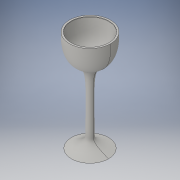
# Autodesk Inventor part: Wine Glass Placeholder
Saved by Autodesk Inventor 2016 (Build 200138000, 138)
## iProperties
Created: 2017-10-31
Part Number: Wine Glass Placeholder
Material: Generic
Document SubType Name: Modeling
Designer: mathaetaes
Density: 1 g/cm^3
Appearance: Default
Author: mathaetaes
Autodesk Inventor part; units mm, degrees
ref_plane "YZ Plane" through (0, 0, 0) normal (1, 0, 0) x (0, 1, 0)
ref_plane "XZ Plane" through (0, 0, 0) normal (0, 1, 0) x (-1, 0, 0)
ref_plane "XY Plane" through (0, 0, 0) normal (0, 0, 1) x (1, 0, 0)
sketch "Sketch2" plane through (0, 0, 0) normal (0, 0, 1) x (1, 0, 0)
  line L0 (34.925, 0) -> (6.35, 11.4298) construction
  line L1 (6.35, 11.4298) -> (6.35, 18.3092) construction
  line L2 (6.35, 18.3092) -> (6.35, 36.1893) construction
  line L3 (6.35, 36.1893) -> (4.3576, 138.0598) construction
  line L4 (4.3576, 138.0598) -> (12.2352, 131.3941) construction
  line L5 (12.2352, 131.3941) -> (40.8943, 150.2751) construction
  line L6 (40.8943, 150.2751) -> (38.7262, 190.0987) construction
  spline S0 degree 4 poles (34.925, 0) (6.35, 11.4298) (6.35, 18.3092) (6.35, 36.1893) (4.3576, 138.0598) (12.2352, 131.3941) (40.8943, 150.2751) (38.7262, 190.0987) knots 1 1 1 1 1 2 3 4 5 5 5 5 5
  line L7 (0, -41.1386) -> (0, 233.3749) projected
  line L8 (32.5436, 0) -> (0, 0) construction
  line L9 (0, 0) -> (0, 28.1933) construction
  line L10 (0, 28.1933) -> (0, 145.2928) construction
  line L11 (0, 145.2928) -> (16.7998, 130.9324) construction
  line L12 (16.7998, 130.9324) -> (28.7084, 150.8624) construction
  line L13 (28.7084, 150.8624) -> (34.5536, 159.8994) construction
  line L14 (34.5536, 159.8994) -> (35.6023, 189.0493) construction
  spline S1 degree 4 poles (32.5436, 0) (0, 0) (0, 28.1933) (0, 145.2928) (16.7998, 130.9324) (28.7084, 150.8624) (34.5536, 159.8994) (35.6023, 189.0493) knots 1 1 1 1 1 2 3 4 5 5 5 5 5
  line L15 (32.5436, 0) -> (34.925, 0)
  line L16 (38.7262, 190.0987) -> (35.6023, 190.0987)
  line L17 (35.6023, 190.0987) -> (35.6023, 189.0493)
  dimension "d7" = 6.35
  constraints: 6 end point, 4 vertical, 2 horizontal, 2 point on line, 1 coincident, 1 perpendicular, 6 other
  measures "d7" distance from line of L2.end L7
revolve "Revolution1" add sketch "Sketch2" angle 360 about axis through (0, -10, 0) along (0, 1, 0)
body "Solid1"
